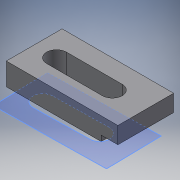
# Autodesk Inventor part: ChipClip
Saved by Autodesk Inventor 2019 (Build 230136000, 136)
## iProperties
Created: 2019-08-13
Part Number: ChipClip
Material: Generic
Document SubType Name: Modeling
Designer: aorfi
Density: 1 g/cm^3
Appearance: Default
Author: aorfi
Autodesk Inventor part; units mm, degrees
ref_plane "YZ Plane" through (0, 0, 0) normal (1, 0, 0) x (0, 1, 0)
ref_plane "XZ Plane" through (0, 0, 0) normal (0, 1, 0) x (-1, 0, 0)
ref_plane "XY Plane" through (0, 0, 0) normal (0, 0, 1) x (1, 0, 0)
sketch "Sketch1" plane through (0, 0, 0) normal (0, 1, 0) x (-1, 0, 0)
  line L0 (4, 2.5) -> (-4, 2.5)
  line L1 (-4, 2.5) -> (-4, -2.5)
  line L2 (-4, -2.5) -> (4, -2.5)
  line L3 (4, -2.5) -> (4, 2.5)
  line L4 (4, 2.5) -> (-4, -2.5) construction
  line L5 (-4, 2.5) -> (4, -2.5) construction
  circle A0 centre (2, 0) radius 0.889
  circle A1 centre (-1, 0) radius 0.889
  line L6 (2, -0.889) -> (-1, -0.889)
  line L7 (2, 0.889) -> (-1, 0.889)
  point P0 (0, 0)
  point P1 (0, 0)
  point P2 (0, 0)
  point P3 (0, 0)
  dimension "d19" = 8
  dimension "d20" = 5
  dimension "d21" = 1.778
  dimension "d22" = 2
  dimension "d23" = 3
  constraints: 16 end point, 4 midpoint, 4 point on circle, 3 parallel, 2 centre point, 2 horizontal, 2 horizontal alignment, 2 tangent, 1 coincident, 1 equal radius, 1 perpendicular
  measures "d19" distance of L1.end L2.end
  measures "d20" distance of L0.end L1.end
  measures "d21" diameter of A0
  measures "d22" distance from line of A0.centre L3
  measures "d23" distance from line of L1 A1.centre
extrude "Extrusion1" add sketch "Sketch1" along normal mid plane 2
sketch "Sketch4" plane through (-4, 1, 2.5) normal (0, 0, 1) x (1, 0, 0)
  line L0 (8, -2) -> (6.5, -2)
  line L1 (6.5, -2) -> (6.5, -1.5)
  line L2 (6.5, -1.5) -> (8, -1.5)
  line L3 (8, -1.5) -> (8, -2)
  line L4 (8, -2) -> (0, -2) projected
  line L5 (8, -2) -> (8, 0) projected
  point P0 (4, -1)
  dimension "d24" = 0.5
  dimension "d25" = 1.5
  constraints: 8 end point, 2 collinear, 2 parallel, 1 horizontal, 1 perpendicular
  measures "d24" distance of L2.end L0.start
  measures "d25" distance of L0.start L0.end
extrude "Extrusion3" cut sketch "Sketch4" against normal through all
fillet "Fillet2" radius 0.5 4 edges at (-4, 0, 2.5) (-4, 0, -2.5) (4, 0.25, 2.5) (4, 0.25, -2.5)
body "Solid1"
